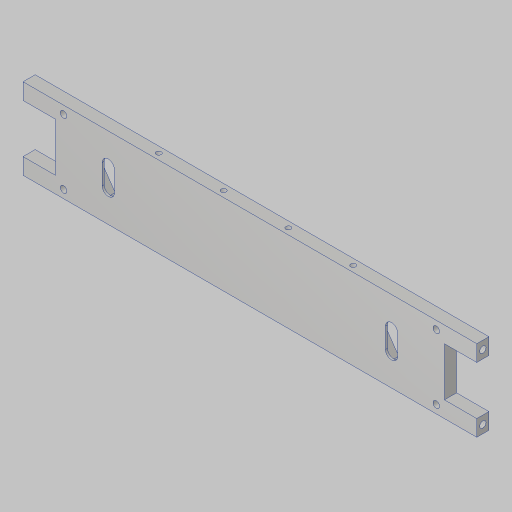
# Autodesk Inventor part: EL2-003
Saved by Autodesk Inventor 2023.5 (Build 275446000, 446)
## iProperties
Created: 2025-01-10
Part Number: EL2-003
Material: Aluminum 6061
Document SubType Name: Modeling
Designer: mavericks
Density: 2.7 g/cm^3
Appearance: Aluminum - Flat
Author: mavericks
Autodesk Inventor part; units mm, degrees
ref_plane "YZ Plane" through (0, 0, 0) normal (1, 0, 0) x (0, 1, 0)
ref_plane "XZ Plane" through (0, 0, 0) normal (0, 1, 0) x (-1, 0, 0)
ref_plane "XY Plane" through (0, 0, 0) normal (0, 0, 1) x (1, 0, 0)
sketch "Sketch1" plane through (0, 0, 0) normal (0, 0, 1) x (1, 0, 0)
  line L0 (-177.8, -31.75) -> (177.8, -31.75)
  line L1 (177.8, -31.75) -> (177.8, 31.75)
  line L2 (177.8, 31.75) -> (-177.8, 31.75)
  line L3 (-177.8, 31.75) -> (-177.8, -31.75)
  line L4 (-177.8, -31.75) -> (177.8, 31.75) construction
  line L5 (177.8, -31.75) -> (-177.8, 31.75) construction
  point P0 (0, 0)
  dimension "d0" = 355.6
  dimension "d1" = 63.5
  constraints: 12 end point, 2 midpoint, 2 parallel, 1 horizontal, 1 perpendicular
  measures "d0" distance of L2.end L1.end
  measures "d1" distance of L1.end L0.end
extrude "Extrusion1" add sketch "Sketch1" along normal blind 9.525
sketch "Sketch5" plane through (177.8, -31.75, 0) normal (1, 0, 0) x (0, 0, -1)
  line L0 (0, 63.5) -> (-9.525, 63.5) construction
  line L1 (-4.7625, 57.15) -> (-4.7625, 6.35) construction
  line L2 (0, 0) -> (0, 63.5) construction
  point P0 (0, 31.75)
  point P1 (-4.7625, 63.5)
  point P2 (-4.7625, 31.75)
  point P3 (0, 31.75)
  dimension "d29" = 50.8
  constraints: 3 midpoint, 2 end point, 2 vertical alignment, 1 horizontal alignment, 1 vertical
  measures "d29" distance of L1.start L1.end
hole "Hole3" at (177.8, 25.4, 4.7625) at (177.8, -25.4, 4.7625) direction (-1, 0, 0) diameter 4.9784 depth 25.4 tip angle 118 thread size "1/4-20 UNC" class "2B" standard "ANSI Unified Screw Threads"
sketch "Sketch6" plane through (-177.8, -31.75, 0) normal (-1, 0, 0) x (0, 0, 1)
  line L0 (0, 63.5) -> (9.525, 63.5) construction
  line L1 (4.7625, 57.15) -> (4.7625, 6.35) construction
  point P0 (0, 31.75)
  point P1 (4.7625, 63.5)
  point P2 (4.7625, 31.75)
  dimension "d37" = 50.8
  constraints: 2 end point, 2 midpoint, 2 vertical alignment, 1 horizontal alignment, 1 vertical
  measures "d37" distance of L1.start L1.end
hole "Hole4" at (-177.8, 25.4, 4.7625) at (-177.8, -25.4, 4.7625) direction (1, 0, 0) diameter 4.3434 depth 25.4 tip angle 118 thread size "12-24 UNC" class "2B" standard "ANSI Unified Screw Threads"
sketch "Sketch8" plane through (0, 0, 9.525) normal (0, 0, 1) x (1, 0, 0)
  line L0 (-152.4, 19.05) -> (-177.8, 19.05)
  line L1 (-177.8, 19.05) -> (-177.8, -19.05)
  line L2 (-177.8, -19.05) -> (-152.4, -19.05)
  line L3 (-152.4, -19.05) -> (-152.4, 19.05)
  line L4 (-152.4, 19.05) -> (-177.8, -19.05) construction
  line L5 (-177.8, 19.05) -> (-152.4, -19.05) construction
  line L6 (177.8, 31.75) -> (-177.8, 31.75) projected
  line L7 (-177.8, 31.75) -> (-177.8, -31.75) projected
  line L8 (177.8, 19.05) -> (152.4, 19.05)
  line L9 (152.4, 19.05) -> (152.4, -19.05)
  line L10 (152.4, -19.05) -> (177.8, -19.05)
  line L11 (177.8, -19.05) -> (177.8, 19.05)
  line L12 (177.8, 19.05) -> (152.4, -19.05) construction
  line L13 (152.4, 19.05) -> (177.8, -19.05) construction
  line L14 (177.8, -31.75) -> (177.8, 31.75) projected
  point P0 (0, 0)
  point P1 (-165.1, 0)
  point P2 (165.1, 0)
  dimension "d45" = 25.4
  dimension "d46" = 38.1
  dimension "d47" = 12.7
  dimension "d49" = 25.4
  dimension "d50" = 38.1
  dimension "d52" = 12.7
  constraints: 24 end point, 4 midpoint, 4 parallel, 2 horizontal, 2 perpendicular, 2 point on line
  measures "d45" distance of L2.end L1.end
  measures "d46" distance of L0.end L1.end
  measures "d47" distance between parallel lines of L6 L0
  measures "d49" distance of L10.end L9.end
  measures "d50" distance of L9.end L8.end
  measures "d52" distance between parallel lines of L6 L8
extrude "Extrusion3" cut sketch "Sketch8" against normal blind 39.6875
sketch "Sketch9" plane through (0, 0, 9.525) normal (0, 0, 1) x (1, 0, 0)
  line L0 (110.998, 7.9375) -> (110.998, -7.9375) construction
  line L1 (106.2355, 7.9375) -> (106.2355, -7.9375)
  line L2 (115.7605, -7.9375) -> (115.7605, 7.9375)
  arc A0 (115.7605, 7.9375) -> (106.2355, 7.9375) centre (110.998, 7.9375) ccw
  arc A1 (106.2355, -7.9375) -> (115.7605, -7.9375) centre (110.998, -7.9375) ccw
  line L3 (-152.4, -19.05) -> (-177.8, -19.05) construction
  line L4 (-177.8, -19.05) -> (-177.8, -31.75) construction
  line L5 (-177.8, -31.75) -> (177.8, -31.75) construction
  line L6 (177.8, -31.75) -> (177.8, -19.05) construction
  line L7 (177.8, -19.05) -> (152.4, -19.05) construction
  line L8 (152.4, -19.05) -> (152.4, 19.05) construction
  line L9 (152.4, 19.05) -> (177.8, 19.05) construction
  line L10 (177.8, 19.05) -> (177.8, 31.75) construction
  line L11 (177.8, 31.75) -> (-177.8, 31.75) construction
  line L12 (-177.8, 31.75) -> (-177.8, 19.05) construction
  line L13 (-177.8, 19.05) -> (-152.4, 19.05) construction
  line L14 (-152.4, 19.05) -> (-152.4, -19.05) construction
  line L15 (0, 0) -> (0, 31.75) construction
  line L16 (-110.998, 7.9375) -> (-110.998, -7.9375) construction
  line L17 (-106.2355, 7.9375) -> (-106.2355, -7.9375)
  line L18 (-115.7605, -7.9375) -> (-115.7605, 7.9375)
  arc A2 (-106.2355, 7.9375) -> (-115.7605, 7.9375) centre (-110.998, 7.9375) ccw
  arc A3 (-115.7605, -7.9375) -> (-106.2355, -7.9375) centre (-110.998, -7.9375) ccw
  line L19 (-177.8, -31.75) -> (-177.8, -19.05) construction
  line L20 (-177.8, -19.05) -> (-152.4, -19.05) construction
  line L21 (-152.4, -19.05) -> (-152.4, 19.05) construction
  line L22 (-152.4, 19.05) -> (-177.8, 19.05) construction
  circle A4 centre (-139.7, 0) radius 1.9812 construction
  circle A5 centre (-139.7, -25.4) radius 1.9812 construction
  point P0 (110.998, 0)
  point P1 (110.998, -12.7)
  point P2 (110.998, 12.7)
  point P3 (-110.998, 0)
  point P4 (-110.998, -12.7)
  point P5 (-110.998, 12.7)
  point P6 (-139.7, 25.4)
  dimension "d55" = 9.525
  dimension "d56" = 25.4
  dimension "d57" = 66.802
  constraints: 26 end point, 10 point on circle, 9 symmetric about line, 6 centre point, 4 tangent, 2 midpoint, 1 parallel, 1 vertical, 2 other
  measures "d55" diameter of A1
  measures "d56" distance of point (110.998, -12.7) point (110.998, 12.7)
  measures "d57" horizontal distance of L5.end point (110.998, 0)
extrude "Extrusion4" cut sketch "Sketch9" against normal through all
sketch "Sketch10" plane through (-177.8, 31.75, 0) normal (0, 1, 0) x (1, 0, 0)
  line L0 (355.6, 0) -> (0, 0) construction
  line L1 (0, 0) -> (0, -9.525) construction
  line L2 (355.6, -9.525) -> (0, -9.525) construction
  line L3 (355.6, 0) -> (355.6, -9.525) construction
  line L4 (0, 0) -> (0, -9.525) construction
  line L5 (177.8, 0) -> (177.8, -9.525) construction
  line L6 (0, -9.525) -> (355.6, -9.525) construction
  point P0 (101.6, -4.7625)
  point P1 (152.4, -4.7625)
  point P2 (0, -4.7625)
  point P3 (0, -4.7625)
  point P4 (254, -4.7625)
  point P5 (203.2, -4.7625)
  dimension "d60" = 101.6
  dimension "d61" = 50.8
  constraints: 3 midpoint, 2 end point, 2 horizontal alignment, 2 symmetric about line
  measures "d60" distance of point (0, -4.763) point (101.6, -4.763)
  measures "d61" distance of point (152.4, -4.763) point (101.6, -4.763)
sketch "Sketch11" plane through (0, 0, 0) normal (0, 0, 1) x (1, 0, 0)
  line L0 (27.3812, -31.75) -> (23.4188, -31.75) projected
  line L1 (-23.4188, -31.75) -> (-27.3812, -31.75) projected
  line L2 (115.7605, 7.9375) -> (115.7605, -7.9375) construction
  arc A0 (106.2355, -7.9375) -> (115.7605, -7.9375) centre (110.998, -7.9375) ccw construction
  line L3 (106.2355, -7.9375) -> (106.2355, 7.9375) construction
  arc A1 (115.7605, 7.9375) -> (106.2355, 7.9375) centre (110.998, 7.9375) ccw construction
  arc A2 (-106.2355, 7.9375) -> (-115.7605, 7.9375) centre (-110.998, 7.9375) ccw construction
  line L4 (-106.2355, 7.9375) -> (-106.2355, -7.9375) construction
  arc A3 (-115.7605, -7.9375) -> (-106.2355, -7.9375) centre (-110.998, -7.9375) ccw construction
  line L5 (-115.7605, -7.9375) -> (-115.7605, 7.9375) construction
  line L6 (-152.4, -19.05) -> (-177.8, -19.05) projected
  line L7 (-177.8, -19.05) -> (-177.8, -31.75) projected
  line L8 (-177.8, -31.75) -> (177.8, -31.75) projected
  line L9 (177.8, -31.75) -> (177.8, -19.05) projected
  line L10 (177.8, -19.05) -> (152.4, -19.05) projected
  line L11 (152.4, -19.05) -> (152.4, 19.05) projected
  line L12 (152.4, 19.05) -> (177.8, 19.05) projected
  line L13 (177.8, 19.05) -> (177.8, 31.75) projected
  line L14 (177.8, 31.75) -> (-177.8, 31.75) projected
  line L15 (-177.8, 31.75) -> (-177.8, 19.05) projected
  line L16 (-177.8, 19.05) -> (-152.4, 19.05) projected
  line L17 (-152.4, 19.05) -> (-152.4, -19.05) projected
  line L18 (-78.1812, -31.75) -> (-78.1812, -31.75) projected
  line L19 (-146.05, 25.4) -> (146.05, 25.4) construction
  line L20 (146.05, 25.4) -> (146.05, -25.4) construction
  line L21 (146.05, -25.4) -> (-146.05, -25.4) construction
  line L22 (-146.05, -25.4) -> (-146.05, 25.4) construction
  line L23 (-110.998, 25.4) -> (-76.2, -25.4) construction
  line L24 (-76.2, -25.4) -> (-25.4, 25.4) construction
  line L25 (-25.4, 25.4) -> (25.4, -25.4) construction
  line L26 (25.4, -25.4) -> (76.2, 25.4) construction
  line L27 (76.2, 25.4) -> (110.998, -25.4) construction
  line L28 (110.998, -25.4) -> (146.05, 25.4) construction
  line L29 (-111.252, -25.4) -> (-76.2, 25.4) construction
  line L30 (-76.2, 25.4) -> (-25.4, -25.4) construction
  line L31 (-25.4, -25.4) -> (25.4, 25.4) construction
  line L32 (25.4, 25.4) -> (76.2, -25.4) construction
  line L33 (76.2, -25.4) -> (111.252, 25.4) construction
  line L34 (146.05, -25.4) -> (111.252, 25.4) construction
  line L35 (-109.3233, -25.4) -> (-75.9754, 22.9303) construction
  line L36 (-75.9754, 22.9303) -> (-25.4, -27.6451) construction
  line L37 (-25.4, -27.6451) -> (25.4, 23.1549) construction
  line L38 (25.4, 23.1549) -> (76.4246, -27.8697) construction
  line L39 (76.4246, -27.8697) -> (111.2472, 22.5978) construction
  line L40 (111.2472, 22.5978) -> (144.1258, -25.4) construction
  line L41 (-113.1807, -25.4) -> (-76.4246, 27.8697) construction
  line L42 (-76.4246, 27.8697) -> (-25.4, -23.1549) construction
  line L43 (-25.4, -23.1549) -> (25.4, 27.6451) construction
  line L44 (25.4, 27.6451) -> (75.9754, -22.9303) construction
  line L45 (75.9754, -22.9303) -> (111.2568, 28.2022) construction
  line L46 (111.2568, 28.2022) -> (146.05, -22.5909) construction
  line L47 (-109.0738, 25.4) -> (-75.9707, -22.9256) construction
  line L48 (-75.9707, -22.9256) -> (-25.4, 27.6451) construction
  line L49 (-25.4, 27.6451) -> (25.4, -23.1549) construction
  line L50 (25.4, -23.1549) -> (76.4293, 27.8744) construction
  line L51 (76.4293, 27.8744) -> (111.0028, -22.5978) construction
  line L52 (111.0028, -22.5978) -> (144.1213, 25.4) construction
  line L53 (-112.9222, 25.4) -> (-76.4293, -27.8744) construction
  line L54 (-76.4293, -27.8744) -> (-25.4, 23.1549) construction
  line L55 (-25.4, 23.1549) -> (25.4, -27.6451) construction
  line L56 (25.4, -27.6451) -> (75.9707, 22.9256) construction
  line L57 (75.9707, 22.9256) -> (110.9932, -28.2022) construction
  line L58 (110.9932, -28.2022) -> (146.05, 22.6047) construction
  line L59 (-111.252, -25.4) -> (-146.05, 25.4) construction
  line L60 (-110.998, 25.4) -> (-146.05, -25.4) construction
  line L61 (-144.1213, 25.4) -> (-109.3233, -25.4) construction
  line L62 (-146.05, 22.5909) -> (-113.1762, -25.4) construction
  line L63 (-144.1258, -25.4) -> (-109.0738, 25.4) construction
  line L64 (-146.05, -22.6047) -> (-112.9267, 25.4) construction
  line L65 (-146.05, 25.4) -> (146.05, 25.4)
  line L66 (146.05, 25.4) -> (146.05, -25.4)
  line L67 (146.05, -25.4) -> (-146.05, -25.4)
  line L68 (-146.05, -25.4) -> (-146.05, 25.4)
  line L69 (-146.05, 22.5909) -> (-113.1762, -25.4)
  line L70 (-109.3233, -25.4) -> (-75.9754, 22.9303)
  line L71 (-75.9754, 22.9303) -> (-27.6451, -25.4)
  line L72 (-23.1549, -25.4) -> (25.4, 23.1549)
  line L73 (25.4, 23.1549) -> (73.9549, -25.4)
  line L74 (78.1287, -25.4) -> (111.2472, 22.5978)
  line L75 (111.2472, 22.5978) -> (144.1258, -25.4)
  line L76 (146.05, -22.5909) -> (113.1762, 25.4)
  line L77 (109.3233, 25.4) -> (75.9754, -22.9303)
  line L78 (75.9754, -22.9303) -> (27.6451, 25.4)
  line L79 (23.1549, 25.4) -> (-25.4, -23.1549)
  line L80 (-25.4, -23.1549) -> (-73.9549, 25.4)
  line L81 (-78.1287, 25.4) -> (-111.245, -22.5946)
  line L82 (-111.245, -22.5946) -> (-144.1213, 25.4)
  line L83 (-144.1258, -25.4) -> (-111.005, 22.6011)
  line L84 (-111.005, 22.6011) -> (-78.1242, -25.4)
  line L85 (-73.9549, -25.4) -> (-25.4, 23.1549)
  line L86 (-25.4, 23.1549) -> (23.1549, -25.4)
  line L87 (27.6451, -25.4) -> (75.9707, 22.9256)
  line L88 (75.9707, 22.9256) -> (109.0738, -25.4)
  line L89 (112.9267, -25.4) -> (146.05, 22.6047)
  line L90 (144.1213, 25.4) -> (111.0028, -22.5978)
  line L91 (78.1242, 25.4) -> (111.0028, -22.5978)
  line L92 (73.9549, 25.4) -> (25.4, -23.1549)
  line L93 (25.4, -23.1549) -> (-23.1549, 25.4)
  line L94 (-27.6451, 25.4) -> (-75.9707, -22.9256)
  line L95 (-75.9707, -22.9256) -> (-109.0738, 25.4)
  line L96 (-112.9267, 25.4) -> (-146.05, -22.6047)
  point P0 (0, 0)
  point P1 (-128.5807, 2.7131)
  point P2 (-128.5947, -2.8912)
  point P3 (-113.1762, -25.4)
  point P4 (-130.5142, -0.0891)
  point P5 (128.5925, 2.8945)
  point P6 (130.5142, 0.0891)
  point P7 (128.583, -2.7098)
  point P8 (93.6575, -2.8945)
  point P9 (95.5887, -0.0956)
  point P10 (126.6613, 0.0956)
  point P11 (93.667, 2.7098)
  point P12 (91.7358, -0.0891)
  point P13 (53.0451, 0)
  point P14 (50.8, 2.2451)
  point P15 (50.8, -2.2451)
  point P16 (2.2451, 0)
  point P17 (48.5549, 0)
  point P18 (0, -2.2451)
  point P19 (0, 2.2451)
  point P20 (-2.2451, 0)
  point P21 (-48.5549, 0)
  point P22 (-50.8, 2.2451)
  point P23 (-50.8, -2.2451)
  point P24 (-93.667, -2.7098)
  point P25 (-91.7358, 0.0891)
  point P26 (-53.0451, 0)
  point P27 (-93.6575, 2.8945)
  point P28 (-95.5887, 0.0956)
  point P29 (-126.6612, -0.0891)
  point P30 (0, 0)
  dimension "d69" = 6.35
  dimension "d72" = 1.5875
  dimension "d73" = 1.5875
  dimension "d74" = 1.5875
  dimension "d75" = 1.5875
  dimension "d76" = 1.5875
  dimension "d77" = 1.5875
  dimension "d81" = 41.1528
  constraints: 151 end point, 31 point on line, 16 perpendicular, 14 parallel, 8 collinear, 2 midpoint, 1 coincident, 1 vertical, 1 vertical alignment, 81 other
  measures "d72" distance between parallel lines of L29 L35
  measures "d73" distance between parallel lines of L29 L41
  measures "d74" distance between parallel lines of L23 L47
  measures "d75" distance between parallel lines of L23 L53
  measures "d76" distance between parallel lines of L60 L64
  measures "d77" distance between parallel lines of L59 L62
  measures "d81" distance from line of L11 L39.end
extrude "Extrusion5" cut sketch "Sketch11" along normal blind 7.9375 contours L65 L96 L82 | L69 L96 L68 | L65 L81 L95 | L83 L84 L81 L82 | L69 L67 L83 | L65 L94 L80 | L70 L71 L94 L95 | L70 L84 L67 | L65 L79 L93 | L85 L86 L79 L80 | L85 L71 L67 | L65 L92 L78 | L72 L73 L92 L93 | L72 L86 L67 | L65 L77 L91 | L87 L88 L77 L78 | L87 L73 L67 | L65 L90 L76 | L74 L75 L90 L91 | L74 L88 L67 | L89 L66 L76 | L89 L75 L67
fillet "Fillet1" radius 4.7625 72 edges at (-53.0451, 0, 3.9688) (-91.7358, 0.0891, 3.9688) (-48.5549, 0, 3.9688) (-2.2451, 0, 3.9688) (50.8, -2.2451, 3.9688) (27.6451, -25.4, 3.9688) (73.9549, -25.4, 3.9688) (95.5887, -0.0956, 3.9688) (111.0028, -22.5978, 3.9688) (111.2472, 22.5978, 3.9688) (126.6613, 0.0956, 3.9688) (128.5925, 2.8945, 3.9688) (144.1213, 25.4, 3.9688) (113.1762, 25.4, 3.9688) (-128.5807, 2.7131, 3.9688) (-112.9267, 25.4, 3.9688) (-144.1213, 25.4, 3.9688) (146.05, 22.6047, 3.9688) (130.5142, 0.0891, 3.9688) (146.05, -22.5909, 3.9688) (109.3233, 25.4, 3.9688) (93.667, 2.7098, 3.9688) (48.5549, 0, 3.9688) (2.2451, 0, 3.9688) (-50.8, 2.2451, 3.9688) (-27.6451, 25.4, 3.9688) (-73.9549, 25.4, 3.9688) (-93.6575, 2.8945, 3.9688) (-109.0738, 25.4, 3.9688) (-109.3233, -25.4, 3.9688) (-93.667, -2.7098, 3.9688) (-23.1549, 25.4, 3.9688) (0, 2.2451, 3.9688) (23.1549, 25.4, 3.9688) (50.8, 2.2451, 3.9688) (73.9549, 25.4, 3.9688) (27.6451, 25.4, 3.9688) (93.6575, -2.8945, 3.9688) (109.0738, -25.4, 3.9688) (-146.05, -22.6047, 3.9688) (-130.5142, -0.0891, 3.9688) (-146.05, 22.5909, 3.9688) (-128.5947, -2.8912, 3.9688) (-144.1258, -25.4, 3.9688) (-113.1762, -25.4, 3.9688) (128.583, -2.7098, 3.9688) (112.9267, -25.4, 3.9688) (144.1258, -25.4, 3.9688) (53.0451, 0, 3.9688) (91.7358, -0.0891, 3.9688) (23.1549, -25.4, 3.9688) (0, -2.2451, 3.9688) (-23.1549, -25.4, 3.9688) (-50.8, -2.2451, 3.9688) (-73.9549, -25.4, 3.9688) (-27.6451, -25.4, 3.9688) (-95.5887, 0.0956, 3.9688) (-111.005, 22.6011, 3.9688) (-111.245, -22.5946, 3.9688) (-126.6612, -0.0891, 3.9688) (78.1242, 25.4, 3.9688) (75.9707, 22.9256, 3.9688) (25.4, 23.1549, 3.9688) (-25.4, 23.1549, 3.9688) (-75.9754, 22.9303, 3.9688) (-75.9707, -22.9256, 3.9688) (-78.1242, -25.4, 3.9688) (-78.1287, 25.4, 3.9688) (-25.4, -23.1549, 3.9688) (25.4, -23.1549, 3.9688) (75.9754, -22.9303, 3.9688) (78.1287, -25.4, 3.9688)
hole "Hole6" at (-76.2, 31.75, 4.7625) at (-25.4, 31.75, 4.7625) at (76.2, 31.75, 4.7625) at (25.4, 31.75, 4.7625) direction (0, -1, 0) diameter 3.9624 end through all thread size "10-32 UNF" class "2B" standard "ANSI Unified Screw Threads"
sketch "Sketch12" plane through (0, 0, 0) normal (0, 0, -1) x (-1, 0, 0)
  line L0 (-177.8, 19.05) -> (-177.8, 31.75) projected
  line L1 (-177.8, -31.75) -> (-177.8, -19.05) projected
  line L2 (177.8, 31.75) -> (177.8, 19.05) projected
  point P0 (0, 0)
  point P1 (-146.05, 25.4)
  point P2 (146.05, 25.4)
  point P3 (146.05, -25.4)
  point P4 (-146.05, -25.4)
  point P5 (-177.8, 25.4)
  point P6 (-177.8, 25.4)
  point P7 (-177.8, -25.4)
  point P8 (177.8, 25.4)
  dimension "d89" = 31.75
  dimension "d90" = 31.75
  constraints: 4 horizontal alignment, 4 midpoint, 2 vertical alignment
  measures "d89" distance of point (-146.05, 25.4) point (-177.8, 25.4)
  measures "d90" distance of point (177.8, 25.4) point (146.05, 25.4)
hole "Hole7" at (146.05, 25.4, 0) at (-146.05, 25.4, 0) at (-146.05, -25.4, 0) at (146.05, -25.4, 0) direction (0, 0, 1) diameter 5.1054 end through all clearance for "Flat Head Machine Screw (82)" size "#10" standard "Ansi Unified Screw Threads"
body "Solid1"
